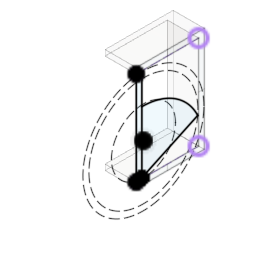
model (Autodesk Fusion 360 design; units mm, degrees)
Autodesk Fusion 360 part; units mm, degrees
sketch "Sketch1" plane through (0, 0, 0) normal (1, 0, 0) x (0, 1, 0) in component "box"
  line L0 (0, 0) -> (200, 0)
  line L1 (200, 0) -> (200, 300)
  line L2 (200, 300) -> (0, 300)
  line L3 (0, 300) -> (0, 0) construction
  line L4 (0, 300) -> (0, 318)
  line L5 (0, 318) -> (218, 318)
  line L6 (218, 318) -> (218, -18)
  line L7 (218, -18) -> (0, -18)
  line L8 (0, -18) -> (0, 0)
  line L9 (100, 300) -> (100, 318) construction
  line L10 (200, 150) -> (218, 150) construction
  line L11 (100, 0) -> (100, -18) construction
  dimension "d8" = 300
  dimension "d9" = 200
  dimension "d10" = 18
  constraint horizontal L0
  constraint vertical L1
  constraint horizontal L2
  constraint vertical L3
  constraint coincident L0.start L3.end
  constraint vertical L4
  constraint horizontal L5
  constraint vertical L6
  constraint horizontal L7
  constraint vertical L8
  constraint midpoint L2 L9.start
  constraint coincident L5 L9.end
  constraint perpendicular L5 L9
  constraint midpoint L1 L10.start
  constraint midpoint L6 L10.end
  constraint perpendicular L6 L10
  constraint midpoint L0 L11.start
  constraint coincident L7 L11.end
  constraint perpendicular L7 L11
  constraint equal L9 L10
  measures "d8" distance of L0.end L1.end
  measures "d9" distance of L0.start L0.end
  measures "d10" distance of L7.end L0.start
extrude "Extrude1" add sketch "Sketch1" against normal blind 100 in component "box"
sketch "Sketch1 (2)" plane through (0, 0, 0) normal (1, 0, 0) x (0, 1, 0) in component "hinge"
  line L0 (0, 297) -> (18, 297)
  line L1 (18, 297) -> (18, 3)
  line L2 (18, 3) -> (0, 3)
  line L3 (0, 3) -> (0, 297)
  line L4 (200, 300) -> (0, 300) construction
  line L5 (0, 0) -> (200, 0) construction
  line L6 (0, 0) -> (0, 3) construction
  line L7 (0, 297) -> (0, 300) construction
  line L8 (18, 3) -> (197, 86.4691)
  arc A0 (197, 86.4691) -> (18, 200.5046) centre (18, 3) ccw
  circle A1 centre (23, 103) radius 5
  circle A2 centre (23, 103) radius 102.6109 construction
  circle A3 centre (23, 103) radius 174.7835 construction
  circle A4 centre (23, 103) radius 194.0644 construction
  dimension "d13" = 3
  dimension "d14" = 18
  dimension "d15" = 3
  dimension "d16" = 10
  dimension "d17" = 5
  dimension "d18" = 100
  dimension "d19" = 65
  constraint horizontal L0
  constraint vertical L1
  constraint horizontal L2
  constraint vertical L3
  constraint coincident L5.start L6.start
  constraint coincident L4.end L7.end
  constraint vertical L7
  constraint equal L6 L7
  constraint coincident L1.end L2.start
  constraint coincident L1 A0.end
  constraint concentric A1 A2
  constraint coincident L2.end A2
  constraint concentric A2 A3
  constraint coincident L8.end A3
  constraint concentric A3 A4
  constraint coincident L0.end A4
  measures "d13" distance of L0.start L4.end
  measures "d14" distance of L0.start L0.end
  measures "d15" horizontal distance of L5.end L8.end
  measures "d16" diameter of A1
  measures "d17" horizontal distance of L1.end A1.centre
  measures "d18" vertical distance of L1.end A1.centre
  measures "d19" angle of L1 L8
component "mechanism" placed x (1, 0, 0) y (0, 1, 0) z (0, 0, 1) at (0, 0, 0)
component "box" placed x (1, 0, 0) y (0, 1, 0) z (0, 0, 1) at (0, 0, 0) in component "mechanism"
component "hinge" placed x (1, 0, 0) y (0, 1, 0) z (0, 0, 1) at (0, 0, 0) in component "mechanism"
equation "d15 = d13"
